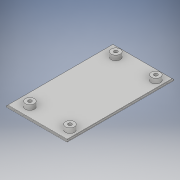
# Autodesk Inventor part: Bottom
Saved by Autodesk Inventor 2019 (Build 230136000, 136)
## iProperties
Created: 2020-10-12
Part Number: Bottom
Material: Generisch
Document SubType Name: Modeling
Designer: d_fel
Density: 1 g/cm^3
Appearance: Vorgabe
Author: d_fel
Autodesk Inventor part; units mm, degrees
ref_plane "YZ Plane" through (0, 0, 0) normal (1, 0, 0) x (0, 1, 0)
ref_plane "XZ Plane" through (0, 0, 0) normal (0, 1, 0) x (-1, 0, 0)
ref_plane "XY Plane" through (0, 0, 0) normal (0, 0, 1) x (1, 0, 0)
sketch "Skizze1" plane through (0, 0, 0) normal (0, 1, 0) x (-1, 0, 0)
  line L0 (0, 0) -> (54.1, 0)
  line L1 (54.1, 0) -> (54.1, -94.74)
  line L2 (54.1, -94.74) -> (0, -94.74)
  line L3 (0, -94.74) -> (0, 0)
  dimension "d0" = 94.74
  dimension "d1" = 54.1
  constraints: 8 end point, 2 parallel, 1 horizontal, 1 perpendicular
  measures "d0" distance of L0.end L1.end
  measures "d1" distance of L1.end L2.end
extrude "Extrusion1" add sketch "Skizze1" along normal blind 1.5
sketch "Skizze2" plane through (0, 1.5, 0) normal (0, 1, 0) x (1, 0, 0)
  line L0 (-54.1, 0) -> (0, 0) projected
  line L1 (0, 94.74) -> (-54.1, 94.74) projected
  line L2 (0, 0) -> (-54.1, 0)
  line L3 (-54.1, 0) -> (-54.1, 94.74)
  line L4 (-54.1, 94.74) -> (0, 94.74)
  line L5 (0, 94.74) -> (0, 0)
  line L6 (-53.35, 93.99) -> (-53.35, 0.75)
  line L7 (-53.35, 0.75) -> (-0.75, 0.75)
  line L8 (-0.75, 0.75) -> (-0.75, 93.99)
  line L9 (-0.75, 93.99) -> (-53.35, 93.99)
  dimension "d4" = 0.75
  constraints: 16 end point, 4 parallel, 2 perpendicular, 1 horizontal, 3 other
  measures "d4" distance between parallel lines of L3 L6
extrude "Extrusion2" cut sketch "Skizze2" against normal blind 0.75
sketch "Skizze3" plane through (0, 1.5, 0) normal (0, 1, 0) x (1, 0, 0)
  circle A0 centre (-42.29, 9.27) radius 4
  circle A1 centre (-42.29, 85.47) radius 4
  circle A2 centre (-6.73, 85.47) radius 4
  circle A3 centre (-6.73, 9.27) radius 4
  line L0 (0, 0) -> (-54.1, 0) projected
  line L1 (-0.75, 0.75) -> (-0.75, 93.99) projected
  line L2 (-53.35, 0.75) -> (-0.75, 0.75) projected
  dimension "d7" = 8
  dimension "d8" = 8
  dimension "d9" = 8
  dimension "d10" = 8
  dimension "d12" = 5.98
  dimension "d13" = 5.98
  dimension "d14" = 35.56
  dimension "d15" = 35.56
  dimension "d16" = 8.52
  dimension "d17" = 76.2
  constraints: 4 centre point, 2 horizontal alignment
  measures "d7" diameter of A3
  measures "d8" diameter of A0
  measures "d9" diameter of A1
  measures "d10" diameter of A2
  measures "d12" distance from line of L1 A3.centre
  measures "d13" distance from line of L1 A2.centre
  measures "d14" distance of A0.centre A3.centre
  measures "d15" distance of A2.centre A1.centre
  measures "d16" distance from line of L2 A3.centre
  measures "d17" distance of A1.centre A0.centre
extrude "Extrusion3" add sketch "Skizze3" along normal blind 4.25
sketch "Skizze4" plane through (-42.29, 5.75, -9.27) normal (0, 1, 0) x (1, 0, 0)
  circle A0 centre (0, 0) radius 4 projected
  circle A1 centre (0, 0) radius 1.55
  circle A2 centre (35.56, 0) radius 4 projected
  circle A3 centre (35.56, 0) radius 1.55
  circle A4 centre (35.56, 76.2) radius 4 projected
  circle A5 centre (35.56, 76.2) radius 1.55
  circle A6 centre (0, 76.2) radius 4 projected
  circle A7 centre (0, 76.2) radius 1.55
  point P0 (42.29, -9.27)
  dimension "d20" = 3.1
  dimension "d21" = 3.1
  dimension "d22" = 3.1
  dimension "d23" = 3.1
  constraints: 4 centre point, 4 coincident
  measures "d20" diameter of A1
  measures "d21" diameter of A3
  measures "d22" diameter of A5
  measures "d23" diameter of A7
extrude "Extrusion4" cut sketch "Skizze4" against normal blind 10 contours A1 | A3 | A5 | A7
sketch "Skizze5" plane through (0, 0, 0) normal (0, -1, 0) x (1, 0, 0)
  circle A0 centre (-6.73, -9.27) radius 1.55 projected
  circle A1 centre (-6.73, -9.27) radius 3
  circle A2 centre (-42.29, -9.27) radius 1.55 projected
  circle A3 centre (-42.29, -9.27) radius 3
  circle A4 centre (-42.29, -85.47) radius 4 projected
  circle A5 centre (-42.29, -85.47) radius 3
  circle A6 centre (-6.73, -85.47) radius 1.55 projected
  circle A7 centre (-6.73, -85.47) radius 3
  point P0 (0, 0)
  dimension "d26" = 6
  dimension "d27" = 6
  dimension "d28" = 6
  dimension "d29" = 6
  constraints: 4 centre point, 4 coincident
  measures "d26" diameter of A1
  measures "d27" diameter of A3
  measures "d28" diameter of A5
  measures "d29" diameter of A7
extrude "Extrusion5" cut sketch "Skizze5" against normal blind 3.5 contours A1 | A3 | A5 | A7
